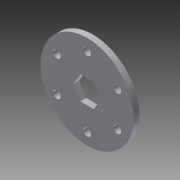
# Autodesk Inventor part: Hex Shaft Connector Pivot
Saved by Autodesk Inventor 2014 (Build 180170000, 170)
## iProperties
Created: 2014-02-11
Part Number: Hex Shaft Connector Pivot
Material: Aluminum 6061
Document SubType Name: Modeling
Designer: Michael
Density: 2.71 g/cm^3
Appearance: Aluminum - Flat
Author: Michael
Autodesk Inventor part; units mm, degrees
ref_plane "YZ Plane" through (0, 0, 0) normal (1, 0, 0) x (0, 1, 0)
ref_plane "XZ Plane" through (0, 0, 0) normal (0, 1, 0) x (-1, 0, 0)
ref_plane "XY Plane" through (0, 0, 0) normal (0, 0, 1) x (1, 0, 0)
sketch "Sketch1" plane through (0, 0, 0) normal (0, 0, 1) x (1, 0, 0)
  circle A0 centre (0, 0) radius 25.4
  circle A1 centre (0, 19.05) radius 2.0828
  line L0 (0, 0) -> (0, 19.05) construction
  circle A2 centre (-16.4978, 9.525) radius 2.0828
  circle A3 centre (-16.4978, -9.525) radius 2.0828
  circle A4 centre (0, -19.05) radius 2.0828
  circle A5 centre (16.4978, -9.525) radius 2.0828
  circle A6 centre (16.4978, 9.525) radius 2.0828
  line L1 (-3.6955, 6.4008) -> (3.6955, 6.4008)
  line L2 (3.6955, 6.4008) -> (7.391, 0)
  line L3 (7.391, 0) -> (3.6955, -6.4008)
  line L4 (3.6955, -6.4008) -> (-3.6955, -6.4008)
  line L5 (-3.6955, -6.4008) -> (-7.391, 0)
  line L6 (-7.391, 0) -> (-3.6955, 6.4008)
  dimension "d0" = 50.8
  dimension "d2" = 4.1656
  dimension "d3" = 19.05
  dimension "d6" = 360
  dimension "d11" = 12.8016
  constraints: 14 end point, 7 centre point, 3 coincident, 1 horizontal, 1 vertical, 26 other
  measures "d0" diameter of A0
  measures "d2" diameter of A1
  measures "d3" distance of L0.end point (0, 0)
  measures "d11" distance between parallel lines of L4 L1
extrude "Extrusion1" add sketch "Sketch1" along normal blind 3.175
body "Solid1"
